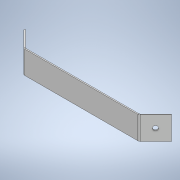
# Autodesk Inventor part: FRONT
Saved by Autodesk Inventor 2020 (Build 240168000, 168)
## iProperties
Created: 2022-07-14
Part Number: FRONT
Material: Generic
Document SubType Name: Sheet Metal
Designer: karimi2
Density: 1 g/cm^3
Sheet Metal Rule: Default_mm
Appearance: Default
Author: karimi2
Autodesk Inventor part; units mm, degrees
ref_plane "YZ Plane" through (0, 0, 0) normal (1, 0, 0) x (0, 1, 0)
ref_plane "XZ Plane" through (0, 0, 0) normal (0, 1, 0) x (-1, 0, 0)
ref_plane "XY Plane" through (0, 0, 0) normal (0, 0, 1) x (1, 0, 0)
sketch "Sketch1" plane through (0, 0, 0) normal (0, 0, 1) x (1, 0, 0)
  line L0 (0, 0) -> (-140, 0)
  line L1 (-140, 0) -> (-140, 40)
  line L2 (-140, 40) -> (0, 40)
  line L3 (0, 0) -> (140, 0)
  line L4 (140, 0) -> (140, 40)
  line L5 (140, 40) -> (0, 40)
  circle A0 centre (-120, 20) radius 4
  circle A1 centre (120, 20) radius 4
  line L6 (-100, 40) -> (-100, 0)
  line L7 (-70, 40) -> (-70, 0)
  line L8 (100, 40) -> (100, 0)
  line L9 (70, 40) -> (70, 0)
  dimension "d0" = 140
  dimension "d1" = 40
  dimension "d51" = 40
  dimension "d52" = 30
  dimension "d53" = 40
  dimension "d54" = 30
  dimension "d55" = 140
  dimension "d56" = 8
  dimension "d57" = 8
  dimension "d58" = 20
  dimension "d59" = 20
  dimension "d60" = 20
  dimension "d61" = 20
  dimension "d62" = 90
  dimension "d63" = 140
  constraints: 20 end point, 4 midpoint, 4 point on line, 3 parallel, 3 perpendicular, 2 centre point, 1 horizontal
  measures "d0" distance of L1.end L2.end
  measures "d1" distance of L0.end L1.end
  measures "d51" distance between parallel lines of L6 L1
  measures "d52" distance between parallel lines of L7 L6
  measures "d53" distance between parallel lines of L4 L8
  measures "d54" distance between parallel lines of L8 L9
  measures "d55" distance from line of L4 L2.end
  measures "d56" diameter of A1
  measures "d57" diameter of A0
  measures "d58" distance from line of L1 A0.centre
  measures "d59" distance from line of A0.centre L0
  measures "d60" distance from line of L3 A1.centre
  measures "d61" distance from line of L4 A1.centre
  measures "d62" angle of L5 L4
  measures "d63" distance from line of L0.start L4
extrude "Plate2" add sketch "Sketch1" along normal blind 2
fold "Fold5" angle 45 bend radius 2 thickness 2 k factor 0.44 line from (-100, 40, 0) to (-100, 0, 0) line at bend centre moving side (-1, 0, 0) folds toward (0, 0, -1)
fold "Fold7" angle 45 bend radius 2 thickness 2 k factor 0.44 line from (100, 40, 0) to (100, 0, 0) line at bend centre moving side (1, 0, 0) folds toward (0, 0, -1)
equation "\"d64\" = Thickness"
equation "\"d65\" = BendReliefWidth"
equation "\"d66\" = BendReliefDepth"
equation "\"d67\" = MinimumRemnant"
equation "\"d68\" = TransitionRadius"
equation "\"d70\" = BendRadius"
equation "\"d77\" = BendReliefWidth"
equation "\"d78\" = BendReliefDepth"
equation "\"d79\" = MinimumRemnant"
equation "\"d80\" = TransitionRadius"
equation "\"d82\" = BendRadius"
equation "\"BendRadius\" = Thickness"
equation "\"BendReliefWidth\" = Thickness"
equation "\"BendReliefDepth\" = 0.5 * Thickness"
equation "\"CornerReliefSize\" = 4 * Thickness"
equation "\"MinimumRemnant\" = 2 * Thickness"
equation "\"TransitionRadius\" = BendRadius"
equation "\"JacobiRadiusSize\" = BendRadius"
equation "\"GapSize\" = Thickness"
equation "\"Thickness\" = 2"
body "Solid2"
